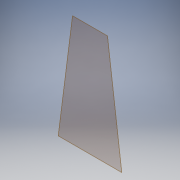
# Autodesk Inventor part: Ramp
Saved by Autodesk Inventor 2018 (Build 220112000, 112)
## iProperties
Created: 2018-09-10
Part Number: Ramp
Material: Generic
Document SubType Name: Modeling
Designer: baoan
Density: 1 g/cm^3
Appearance: Polycarbonate - Smoked
Author: baoan
Autodesk Inventor part; units mm, degrees
ref_plane "YZ Plane" through (0, 0, 0) normal (1, 0, 0) x (0, 1, 0)
ref_plane "XZ Plane" through (0, 0, 0) normal (0, 1, 0) x (-1, 0, 0)
ref_plane "XY Plane" through (0, 0, 0) normal (0, 0, 1) x (1, 0, 0)
sketch "Sketch1" plane through (0, 0, 0) normal (0, 0, 1) x (1, 0, 0)
  line L0 (-254, -444.5) -> (254, -444.5)
  line L1 (-139.7, 444.5) -> (139.7, 444.5)
  line L2 (-139.7, 444.5) -> (-254, -444.5)
  line L3 (254, -444.5) -> (139.7, 444.5)
  line L4 (0, 444.5) -> (0, -444.5) construction
  point P0 (0, 0)
  point P1 (0, 0)
  dimension "d0" = 508
  dimension "d1" = 279.4
  dimension "d2" = 889
  constraints: 10 end point, 3 midpoint, 2 horizontal, 1 coincident, 1 equal length, 1 vertical alignment
  measures "d0" distance of L0.start L0.end
  measures "d1" distance of L1.start L1.end
  measures "d2" distance between parallel lines of L0 L1
extrude "Extrusion1" add sketch "Sketch1" along normal mid plane 3.175
body "Solid1"
